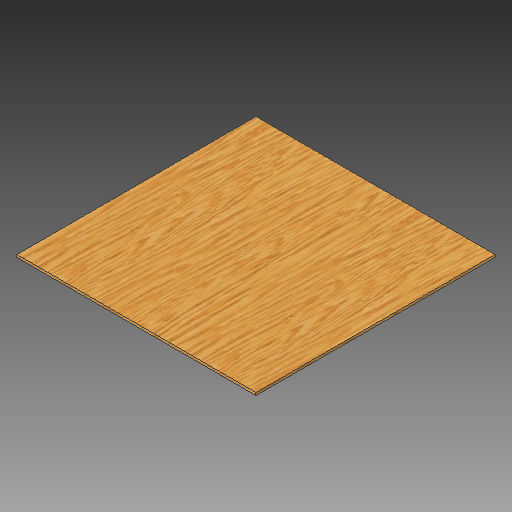
# Autodesk Inventor part: КВ33.044.001
Saved by Autodesk Inventor 2019 (Build 230136000, 136)
## iProperties
Created: 2019-07-15
Part Number: КВ33.044.001
Material: Фанера, финишная
Document SubType Name: Modeling
Designer: user
Density: 0.552 g/cm^3
Appearance: Фанера — новая
Description: Дно
Mass: 2484 g
Surface Area: 11490 cm^2
Volume: 4500 cm^3
Author: user
Autodesk Inventor part; units mm, degrees
ref_plane "YZ Plane" through (0, 0, 0) normal (1, 0, 0) x (0, 1, 0)
ref_plane "XZ Plane" through (0, 0, 0) normal (0, 1, 0) x (-1, 0, 0)
ref_plane "XY Plane" through (0, 0, 0) normal (0, 0, 1) x (1, 0, 0)
sketch "Эскиз1" plane through (0, 0, 0) normal (0, 1, 0) x (-1, 0, 0)
  line L0 (-375, 375) -> (375, 375)
  line L1 (375, 375) -> (375, -375)
  line L2 (375, -375) -> (-375, -375)
  line L3 (-375, -375) -> (-375, 375)
  line L4 (-375, 375) -> (375, -375) construction
  line L5 (375, 375) -> (-375, -375) construction
  point P0 (0, 0)
  dimension "d0" = 750
  dimension "d1" = 750
  constraints: 12 end point, 2 midpoint, 2 parallel, 1 horizontal, 1 perpendicular
  measures "d0" distance of L1.end L2.end
  measures "d1" distance of L0.end L1.end
extrude "Выдавливание1" add sketch "Эскиз1" along normal blind 8
